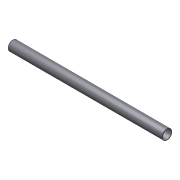
# Autodesk Inventor part: 09R-17.31350
Saved by Autodesk Inventor 2012 (Build 160160000, 160)
## iProperties
Category: PARTsolutions
Created: 2013-01-19
Part Number: 09R-17.31350
Catalog Web Link: www.cadenas.de
Description: Tube - Original Line - Standard Air Cylinders
Document SubType Name: Modeling
Designer: PARTsolutions
Material: Stainless Steel
Mass: 164.183 g
Surface Area: 770.242 cm^2
Volume: 20.3197 cm^3
Density: 8.08 g/cm^3
NB: 09R-17.31350
NN: Tube
NT: Original Line - Standard Air Cylinders
NBSYN: $PN.
LINA: 09R-17.31350
PN: 09R-17.31350
BORE: 1.06250000
BOREPN: 09
MNTALG: '' , 'Front Nose' , 'BF' , 'Front Block' , 'BFT' , 'Front Trunnion' , 'A' , 'Adjustable Stroke'
ACTING: R
ACTINGALG: '' , 'Single Acting' , 'R' , 'Reverse/Double Acting'
NRALG: '' , 'N/A'
L: 17.3135
OD: 1.1130
ODN: 1.1130
ODP: 1.1130
ODB: 1.1410
ID: 1.0715
DV: 0.00000000
LV: 0.00000000
LV1: 0.00000000
G: 0.0300
FOURHOLES: 0
AA: 0.3750
BB: 0.0940
SRALG: 'C' , 'Carbon Steel Rod' , 'SR' , '303 Stainless Steel Rod' , '' , '303 Stainless Steel Rod'
KT: DUMMY
SUPPLIER: Bimba
ARTICLENO: 09R-17.31350
BOMINFO: 09R-17.31350
CREATOR: CADENAS GmbH
PSOL_IDENT_0: {\\10.0.0.242\data_v9\23d-libs\bimba\bimba\bimba_imperial\bimba_full_line\original_line_cylinders\st
PSOL_IDENT_1: andard_air_cylinders\tube.prj},192 {VTYP=3D},{NB=09R-17.31350},{LINA=09R-17.31350},{NN=Tube},{DATE=2
PSOL_IDENT_2: 0.08.2011 07:16:50},{GEOMDATE=18.02.2011 00:00:00},{VERSION=},{LINEID=60},{LINESUBID=-1},{WBVAR=MNT,
PSOL_IDENT_3: ACTING,NR,L,FOURHOLES,SR}  {NB=09R-17.31350},{LINA=09R-17.31350},{KT=DUMMY},{PN=09R-17.31350},{BORE=
PSOL_IDENT_4: 1.06250000},{BOREPN=09},{MNT=},{MNTALG='' , 'Front Nose' , 'BF' , 'Front Block' , 'BFT' , 'Front Tru
PSOL_IDENT_5: nnion' , 'A' , 'Adjustable Stroke'},{ACTING=R},{ACTINGALG= '' , 'Single Acting' , 'R' , 'Reverse/Dou
PSOL_IDENT_6: ble Acting' },{NR=},{NRALG= '' , 'N/A' },{L=17.3135},{OD=1.1130},{ODN=1.1130},{ODP=1.1130},{ODB=1.14
PSOL_IDENT_7: 10},{ID=1.0715},{DV=0.00000000},{LV=0.00000000},{LV1=0.00000000},{G=0.0300},{FOURHOLES=0},{AA=0.3750
PSOL_IDENT_8: },{BB=0.0940},{SR=},{SRALG= 'C' , 'Carbon Steel Rod' , 'SR' , '303 Stainless Steel Rod' , '' , '303
PSOL_IDENT_9: Stainless Steel Rod'}
Title: 09R-17.31350
Author: Cadenas PARTsolutions
Comments: Original Line - Standard Air Cylinders
Autodesk Inventor part; units mm, degrees
sketch "Sketch_1" plane through (0, 0, 0) normal (0, 0, 1) x (1, 0, 0)
  line L0 (439.7629, 0) -> (0, 0)
  arc A0 (-0.6395, 13.2842) -> (-0.6395, 13.1046) centre (-0.5497, 13.1944) ccw
  line L1 (-0.6395, 13.1046) -> (-0.381, 12.846)
  line L2 (-0.381, 12.846) -> (0, 12.846)
  line L3 (0, 12.846) -> (0.762, 13.6081)
  line L4 (0.762, 13.6081) -> (439.0009, 13.6081)
  line L5 (439.0009, 13.6081) -> (439.7629, 12.846)
  line L6 (439.7629, 12.846) -> (440.1439, 12.846)
  line L7 (440.1439, 12.846) -> (440.4024, 13.1046)
  arc A1 (440.4024, 13.1046) -> (440.4024, 13.2842) centre (440.3126, 13.1944) ccw
  line L8 (440.4024, 13.2842) -> (439.7747, 13.9119)
  arc A2 (439.7747, 13.9119) -> (439.2359, 14.1351) centre (439.2359, 13.3731) ccw
  line L9 (439.2359, 14.1351) -> (0.527, 14.1351)
  arc A3 (0.527, 14.1351) -> (-0.0118, 13.9119) centre (0.527, 13.3731) ccw
  line L10 (-0.0118, 13.9119) -> (-0.6395, 13.2842)
  constraints: 22 end point, 8 point on circle, 4 centre point
revolve "Revolution1" add sketch "Sketch_1" angle 360 about axis through (439.7629, 0, 0) along (1, 0, 0)
ref_plane "tube_front_XY" through (0, 0, 0) normal (1, 0, 0) x (0, 0, -1)
ref_plane "tube_front_YZ" through (0, 0, 0) normal (0, 0, -1) x (0, 1, 0)
ref_plane "tube_front_ZX" through (0, 0, 0) normal (0, 1, 0) x (1, 0, 0)
ref_plane "tube_rear_XY" through (439.7629, 0, 0) normal (1, 0, 0) x (0, 0, -1)
ref_plane "tube_rear_YZ" through (439.7629, 0, 0) normal (0, 0, -1) x (0, 1, 0)
ref_plane "tube_rear_ZX" through (439.7629, 0, 0) normal (0, 1, 0) x (1, 0, 0)
ref_plane "cp1_XY" through (219.8815, 14.1351, 0) normal (1, 0, 0) x (0, 0, -1)
ref_plane "cp1_YZ" through (219.8815, 14.1351, 0) normal (0, 0, -1) x (0, 1, 0)
ref_plane "cp1_ZX" through (219.8815, 14.1351, 0) normal (0, 1, 0) x (1, 0, 0)
ref_plane "cp2_XY" through (219.8815, 0, -14.1351) normal (1, 0, 0) x (0, 0, -1)
ref_plane "cp2_YZ" through (219.8815, 0, -14.1351) normal (0, 0, -1) x (0, 1, 0)
ref_plane "cp2_ZX" through (219.8815, 0, -14.1351) normal (0, 1, 0) x (1, 0, 0)
ref_plane "cp3_XY" through (219.8815, -14.1351, 0) normal (1, 0, 0) x (0, 0, -1)
ref_plane "cp3_YZ" through (219.8815, -14.1351, 0) normal (0, 0, -1) x (0, 1, 0)
ref_plane "cp3_ZX" through (219.8815, -14.1351, 0) normal (0, 1, 0) x (1, 0, 0)
ref_plane "cp4_XY" through (219.8815, 0, 14.1351) normal (1, 0, 0) x (0, 0, -1)
ref_plane "cp4_YZ" through (219.8815, 0, 14.1351) normal (0, 0, -1) x (0, 1, 0)
ref_plane "cp4_ZX" through (219.8815, 0, 14.1351) normal (0, 1, 0) x (1, 0, 0)
body "Solid1"
